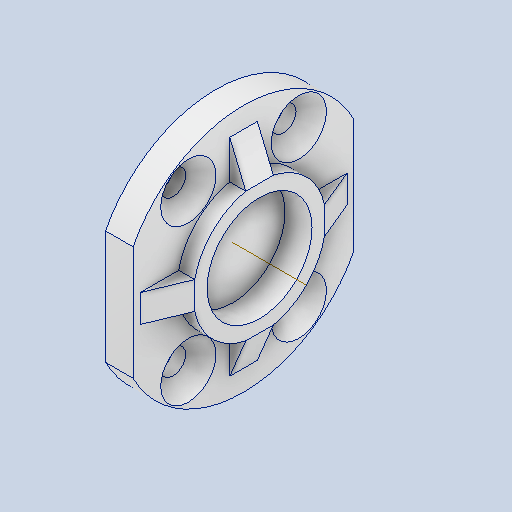
# Autodesk Inventor part: ParallelMecha_DrivenLink_ShaftFixation
Saved by Autodesk Inventor 2022 (Build 260153000, 153)
## iProperties
Created: 2022-08-03
Part Number: ParallelMecha_DrivenLink_ShaftFixation
Material: Aluminium 6061
Document SubType Name: Modeling
Designer: alexw
Density: 2.7 g/cm^3
Appearance: Aluminium - flach
Mass: 19.1726 g
Surface Area: 43.8991 cm^2
Volume: 7.10097 cm^3
DrivenPart_Flansch_TotalThickness: 9,000 mm
FixationHole_Dia: 34,500 mm
Author: alexw
Autodesk Inventor part; units mm, degrees
ref_plane "YZ Plane" through (0, 0, 0) normal (1, 0, 0) x (0, 1, 0)
ref_plane "XZ Plane" through (0, 0, 0) normal (0, 1, 0) x (-1, 0, 0)
ref_plane "XY Plane" through (0, 0, 0) normal (0, 0, 1) x (1, 0, 0)
sketch "Skizze1" plane through (0, 0, 0) normal (0, 0, 1) x (1, 0, 0)
  line L0 (0, 0) -> (0, 22.5)
  line L1 (0, 22.5) -> (5, 22.5)
  line L2 (5, 22.5) -> (5, 12)
  line L3 (5, 12) -> (7.9, 12)
  line L4 (7.9, 12) -> (7.9, 9.5)
  line L5 (7.9, 9.5) -> (3, 9.5)
  line L6 (3, 9.5) -> (3, 0)
  line L7 (3, 0) -> (0, 0)
  line L8 (5, 17.25) -> (0, 17.25) construction
  line L9 (0, 18.75) -> (5, 18.75) construction
  line L10 (0, 15.75) -> (5, 15.75) construction
  line L11 (9, 12) -> (9, 0) construction
  line L12 (5, 12) -> (5, 0) construction
  dimension "d0" = 19
  dimension "d3" = 5
  dimension "d5" = 3
  dimension "d6" = 1.5
  dimension "d7" = 3.75
  dimension "d17" = 2.5
  dimension "d18" = 24
  dimension "d31" = 1.1
  dimension "d32" = 4
  dimension "d33" = 2
  dimension "d34" = 3
  dimension "DrivenPart_Flansch_TotalThickness" = 9
  dimension "d41" = 45
  dimension "FixationHole_Dia" = 34.5
  constraints: 26 end point, 9 perpendicular, 9 point on line, 4 vertical, 1 midpoint
  measures "d0" diameter of L5 L7
  measures "d3" distance between parallel lines of L2 L0
  measures "d5" distance between parallel lines of L9 L10
  measures "d6" distance between parallel lines of L10 L8
  measures "d7" distance between parallel lines of L1 L9
  measures "d17" distance between parallel lines of L3 L5
  measures "d18" diameter of L3 L7
  measures "d31" distance between parallel lines of L4 L11
  measures "d32" distance between parallel lines of L11 L12
  measures "d33" distance between parallel lines of L6 L12
  measures "d34" distance between parallel lines of L0 L6
  measures "DrivenPart_Flansch_TotalThickness" distance between parallel lines of L0 L11
  measures "d41" diameter of L1 L7
  measures "FixationHole_Dia" diameter of L8 L7
revolve "Umdrehung1" add sketch "Skizze1" angle 360 about axis through (3, 0, 0) along (-1, 0, 0)
sketch "Skizze4" plane through (5, 0, 0) normal (1, 0, 0) x (0, -1, 0)
  line L0 (-14.0557, 10) -> (14.0557, 10) construction
  line L1 (14.0557, 10) -> (14.0557, -10) construction
  line L2 (14.0557, -10) -> (-14.0557, -10) construction
  line L3 (-14.0557, -10) -> (-14.0557, 10) construction
  circle A0 centre (0, 0) radius 12 construction
  line L4 (-14.0557, 10) -> (14.0557, -10) construction
  line L5 (14.0557, 10) -> (-14.0557, -10) construction
  circle A1 centre (0, 0) radius 17.25 construction
  arc A2 (-22.5, 0) -> (-22.5, 0) centre (0, 0) ccw construction
  circle A3 centre (0, 0) radius 22.5 construction
  dimension "d40" = 45
  dimension "d43" = 34.5
  dimension "d38" = 20
  dimension "d39" = 24
  constraints: 12 end point, 6 coincident, 2 midpoint, 2 parallel, 1 horizontal, 1 horizontal alignment, 1 perpendicular, 5 other
  measures "d38" distance of L2.end L0.start
  measures "d39" diameter of A0
hole "Bohrung2" at (5, 14.0557, 10) at (5, 14.0557, -10) at (5, -14.0557, 10) at (5, -14.0557, -10) direction (-1, 0, 0) diameter 4.5 end through all countersink diameter 10 countersink angle 90 clearance for "Innensechskant-Senkkopfschraube DIN EN ISO 10642" size "M4" standard "DIN"
sketch "Skizze5" plane through (5, 0, 0) normal (1, 0, 0) x (0, 0, -1)
  circle A0 centre (0, 0) radius 22.5 projected
  circle A1 centre (0, 0) radius 22.5 projected
  line L0 (-20, -10.3078) -> (-20, 10.3078)
  line L1 (20, -10.3078) -> (20, 10.3078)
  point P0 (0, 0)
  dimension "d51" = 40
  constraints: 4 end point, 3 point on circle, 2 parallel, 1 vertical, 2 other
  measures "d51" distance between parallel lines of L0 L1
extrude "Extrusion2" cut sketch "Skizze5" against normal through all contours A0 L1 | L0 A0
sketch "Skizze6" plane through (7.9, 0, 0) normal (1, 0, 0) x (0, 0, -1)
  line L0 (-2.5, 18.7367) -> (2.5, 18.7367)
  line L1 (2.5, 18.7367) -> (2.5, 11.7367)
  line L2 (2.5, 11.7367) -> (-2.5, 11.7367)
  line L3 (-2.5, 11.7367) -> (-2.5, 18.7367)
  line L4 (0, 0) -> (0, 18.7367) construction
  circle A0 centre (0, 0) radius 12 projected
  dimension "d54" = 5
  dimension "d55" = 7
  constraints: 10 end point, 2 parallel, 1 horizontal, 1 midpoint, 1 perpendicular, 1 vertical, 2 other
  measures "d54" distance between parallel lines of L1 L3
  measures "d55" distance between parallel lines of L0 L2
extrude "Extrusion3" add sketch "Skizze6" against normal up to surface (2.9 mm away) contours L0 L1 A0 L3
sketch "Skizze7" plane through (7.9, 11.7367, 2.5) normal (0, 0, 1) x (1, 0, 0)
  line L0 (0, 7) -> (-2.9, 7) projected
  line L1 (0, 0) -> (-2.9, 0) projected
  line L2 (-2.9, 7) -> (0, 0)
  line L3 (0, 7) -> (0, 0) projected
  point P0 (-7.9, -11.7367)
  constraints: 2 end point
extrude "Extrusion4" cut sketch "Skizze7" against normal through all
pattern_circular "Runde Anordnung1" count 4 over 360 about axis through (5.45, 0, 0) along (1, 0, 0) of "Extrusion3", "Extrusion4"
equation "\"d6\" = 0.5 * d5"
equation "\"d43\" = FixationHole_Dia"
